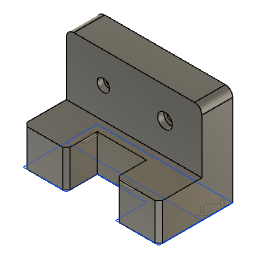
Model 1 v1 (Autodesk Fusion 360 design; units mm, degrees)
Autodesk Fusion 360 part; units mm, degrees
sketch "Sketch1" plane through (0, 0, 0) normal (0, 0, 1) x (1, 0, 0)
  line L0 (15, 30) -> (50, 30)
  line L1 (50, 30) -> (50, 55)
  line L2 (50, 55) -> (90, 55)
  line L3 (90, 55) -> (90, 30)
  line L4 (90, 30) -> (125, 30)
  line L5 (15, 30) -> (15, 90)
  line L6 (125, 30) -> (125, 90)
  line L7 (15, 90) -> (125, 90)
  dimension "d6" = 60
  constraint horizontal L0
  constraint perpendicular L0 L1
  constraint perpendicular L1 L2
  constraint perpendicular L2 L3
  constraint perpendicular L3 L4
  constraint perpendicular L0 L5
  constraint perpendicular L4 L6
  constraint perpendicular L5 L7
  measures "d6" distance of L0.start L5.end
extrude "Extrude1" add sketch "Sketch1" along normal blind 30 makes body 1
chamfer "Chamfer1" distance 3 angle 45 1 edges at (50, 30, 15) on bodies 1
chamfer "Chamfer2" distance 3 angle 45 1 edges at (90, 30, 15) on bodies 1
chamfer "Chamfer3" distance 3 angle 45 1 edges at (125, 30, 15) on bodies 1
chamfer "Chamfer4" distance 3 angle 45 1 edges at (15, 30, 15) on bodies 1
sketch "Sketch2" plane through (0, 0, 0) normal (0, 0, 1) x (1, 0, 0)
  line L0 (15, 90) -> (15, 65)
  line L1 (15, 65) -> (125, 65)
  line L2 (125, 65) -> (125, 90)
  line L3 (125, 90) -> (15, 90)
  constraint vertical L0
  constraint horizontal L1
  constraint perpendicular L1 L2
  constraint perpendicular L2 L3
extrude "Extrude2" add sketch "Sketch2" along normal blind 80 separate body makes body 2
combine "Combine1" operation add target body 1 tool bodies 2
fillet "Fillet1" radius 6 1 edges at (125, 77.5, 80) on bodies 1
fillet "Fillet2" radius 6 1 edges at (15, 77.5, 80) on bodies 1
sketch "Sketch3" plane through (0, 0, 0) normal (0, 1, 0) x (1, 0, 0)
hole "Hole1" at (45, 65, 55) direction (0, 1, 0) diameter 6 depth 25 tip angle 180 counterbore diameter 10 counterbore depth 5 bodies 1
hole "Hole2" at (95, 65, 55) direction (0, 1, 0) diameter 6 depth 25 tip angle 180 counterbore diameter 12 counterbore depth 5 bodies 1
